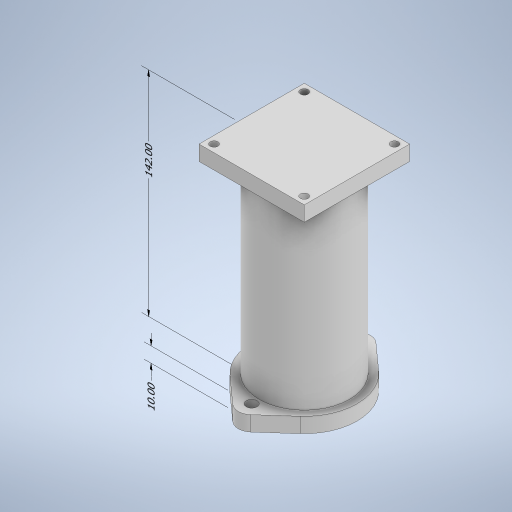
# Autodesk Inventor part: ball-fastening
Saved by Autodesk Inventor 2023 (Build 270158000, 158)
## iProperties
Created: 2024-03-16
Part Number: ball-fastening
Material: Genérico
Document SubType Name: Modeling
Designer: inigo
Density: 1 g/cm^3
Appearance: Valor por defecto
Author: inigo
Autodesk Inventor part; units mm, degrees
ref_plane "YZ Plane" through (0, 0, 0) normal (1, 0, 0) x (0, 1, 0)
ref_plane "XZ Plane" through (0, 0, 0) normal (0, 1, 0) x (-1, 0, 0)
ref_plane "XY Plane" through (0, 0, 0) normal (0, 0, 1) x (1, 0, 0)
sketch "Boceto1" plane through (0, 0, 0) normal (0, 1, 0) x (-1, 0, 0)
  circle A0 centre (0, 0) radius 32.5
  arc A1 (23.3059, -26.112) -> (23.3059, 26.112) centre (0, 0) ccw
  circle A2 centre (0, -35) radius 3.6
  circle A3 centre (0, 0) radius 43.5
  arc A4 (8.153, -31.4608) -> (-5.9184, -41.631) centre (0, -35) ccw
  line L0 (23.3059, -26.112) -> (5.9184, -41.631)
  line L1 (-23.3059, -26.112) -> (-5.9184, -41.631)
  arc A5 (5.9184, -41.631) -> (8.153, -31.4608) centre (0, -35) ccw
  arc A6 (-5.9184, -41.631) -> (5.9184, -41.631) centre (0, -35) ccw
  line L2 (0, 0) -> (19.418, 0)
  circle A7 centre (0, 35) radius 3.6
  arc A8 (-5.9184, 41.631) -> (8.153, 31.4608) centre (0, 35) ccw
  line L3 (23.3059, 26.112) -> (5.9184, 41.631)
  line L4 (-23.3059, 26.112) -> (-5.9184, 41.631)
  arc A9 (8.153, 31.4608) -> (5.9184, 41.631) centre (0, 35) ccw
  arc A10 (5.9184, 41.631) -> (-5.9184, 41.631) centre (0, 35) ccw
  arc A11 (23.3059, 26.112) -> (-23.3059, 26.112) centre (0, 0) ccw
  arc A12 (-23.3059, 26.112) -> (-23.3059, -26.112) centre (0, 0) ccw
  dimension "d0" = 65
  dimension "d2" = 7.2
  dimension "d3" = 87
  constraints: 19 point on circle, 12 centre point, 10 end point, 9 tangent, 7 symmetric about line, 5 coincident, 1 horizontal, 7 other
  measures "d2" diameter of A2
  measures "d3" diameter of A3
extrude "Extrusión1" add sketch "Boceto1" along normal blind 10 contours A0 A4 A8 | A0 A9 A11 A1 L0 A5 | A8 A0 A7 | A0 A7 A11 A9 | A5 A6 A3 A4 A0 A2 | A0 A2 A4 | A8 A11 A7 A0 | A0 A4 L1 A12 A11 A8 | A11 A7 A8 A10 A3 A9 | A9 L3 A11 | A11 L4 A8 | A6 A3 | A3 A10
sketch "Boceto2" plane through (0, 10, 0) normal (0, 1, 0) x (1, 0, 0)
  circle A0 centre (0, 0) radius 30
  dimension "d7" = 60
  constraints: 1 centre point, 1 coincident
  measures "d7" diameter of A0
extrude "Extrusión2" add sketch "Boceto2" along normal blind 122
sketch "Boceto4" plane through (0, 132, 0) normal (0, 1, 0) x (1, 0, 0)
  line L0 (-35, -35) -> (35, -35)
  line L1 (35, -35) -> (35, 35)
  line L2 (35, 35) -> (-35, 35)
  line L3 (-35, 35) -> (-35, -35)
  line L4 (-35, -35) -> (35, 35) construction
  line L5 (35, -35) -> (-35, 35) construction
  line L6 (30, 30) -> (-30, 30)
  line L7 (-30, 30) -> (-30, -30)
  line L8 (-30, -30) -> (30, -30)
  line L9 (30, -30) -> (30, 30)
  line L10 (30, 30) -> (-30, -30) construction
  line L11 (-30, 30) -> (30, -30) construction
  circle A0 centre (-30, 30) radius 2.6
  circle A1 centre (30, 30) radius 2.6
  circle A2 centre (30, -30) radius 2.6
  circle A3 centre (-30, -30) radius 2.6
  point P0 (0, 0)
  dimension "d13" = 70
  dimension "d14" = 70
  dimension "d15" = 60
  dimension "d16" = 5.2
  dimension "d17" = 5.2
  dimension "d18" = 5.2
  dimension "d19" = 5.2
  constraints: 24 end point, 4 centre point, 4 coincident, 4 midpoint, 4 parallel, 2 horizontal, 2 perpendicular, 1 point on line
  measures "d13" distance of L2.end L1.end
  measures "d14" distance of L1.end L0.end
  measures "d15" distance of L7.end L6.end
  measures "d16" diameter of A0
  measures "d17" diameter of A1
  measures "d18" diameter of A2
  measures "d19" diameter of A3
extrude "Extrusión3" add sketch "Boceto4" along normal blind 10 contours L3 L2 L1 L0 | L6 A1 L9 A2 L8 A3 L7 A0
